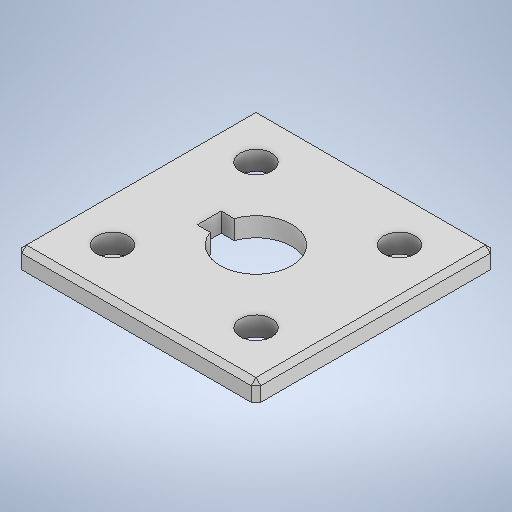
# Autodesk Inventor part: FlanschV1
Saved by Autodesk Inventor 2025.1 (Build 291241000, 241)
## iProperties
Created: 2025-10-12
Part Number: FlanschV1
Material: Generic
Document SubType Name: Modeling
Designer: jonas
Density: 1 g/cm^3
Appearance: Default
Author: jonas
Autodesk Inventor part; units mm, degrees
ref_plane "YZ Plane" through (0, 0, 0) normal (1, 0, 0) x (0, 1, 0)
ref_plane "XZ Plane" through (0, 0, 0) normal (0, 1, 0) x (-1, 0, 0)
ref_plane "XY Plane" through (0, 0, 0) normal (0, 0, 1) x (1, 0, 0)
sketch "Sketch1" plane through (0, 0, 0) normal (0, 1, 0) x (-1, 0, 0)
  line L0 (0, -14.0533) -> (0, 14.0533) construction
  line L1 (4.9803, 0) -> (-4.9803, 0) construction
  line L2 (25, 25) -> (-25, 25)
  line L3 (-25, 25) -> (-25, -25)
  line L4 (-25, -25) -> (25, -25)
  line L5 (25, -25) -> (25, 25)
  arc A0 (7.0711, 2.5) -> (7.0711, -2.5) centre (0, 0) ccw
  line L6 (9.8, 2.5) -> (7.0711, 2.5)
  line L7 (7.0711, -2.5) -> (9.8, -2.5)
  line L8 (9.8, -2.5) -> (9.8, 2.5)
  dimension "d0" = 50
  dimension "d1" = 15
  dimension "d18" = 5
  dimension "d19" = 9.8
  constraints: 18 end point, 3 horizontal, 3 parallel, 3 perpendicular, 2 coincident, 2 midpoint, 2 point on circle, 1 centre point, 1 vertical, 3 other
  measures "d0" distance of L4.end L2.start
  measures "d1" diameter of A0
  measures "d18" distance of L7.end L6.start
  measures "d19" distance from line of L8 point (0, 0)
extrude "Extrusion1" add sketch "Sketch1" along normal blind 4
sketch "Sketch2" plane through (0, 4, 0) normal (0, 1, 0) x (1, 0, 0)
  line L0 (25, 25) -> (-25, 25) projected
  line L1 (-25, 25) -> (-25, -25) projected
  line L2 (-25, -25) -> (25, -25) projected
  line L3 (25, -25) -> (25, 25) projected
  point P0 (0, 0)
  point P1 (-15, -15)
  point P2 (-15, 15)
  point P3 (15, 15)
  point P4 (15, -15)
  dimension "d4" = 10
  dimension "d5" = 10
  dimension "d6" = 10
  dimension "d7" = 10
  constraints: 2 horizontal alignment, 2 vertical alignment
  measures "d4" distance from line of L0 point (-15, 15)
  measures "d5" distance from line of L1 point (-15, 15)
  measures "d6" distance from line of L2 point (15, -15)
  measures "d7" distance from line of L3 point (15, -15)
hole "Hole1" at (-15, 4, 15) at (-15, 4, -15) at (15, 4, -15) at (15, 4, 15) direction (0, -1, 0) diameter 6.6 end through all clearance for "Hex Head Cap Screw DIN EN 24017" size "M6" standard "DIN"
chamfer "Chamfer1" distance 1 angle 45 8 edges at (-25, 2, 25) (25, 2, 25) (25, 2, -25) (0, 4, -25) (-25, 4, 0) (0, 4, 25) (25, 4, 0) (-25, 2, -25)
body "Solid1"
